acrylic_bottom_v20 (Autodesk Fusion 360 design; units mm, degrees)
Autodesk Fusion 360 part; units mm, degrees
sketch "Sketch1" plane through (0, 0, 0) normal (0, 1, 0) x (1, 0, 0)
  line L0 (193.9, 118.363) -> (193.9, 201.7255) construction
  line L1 (23, 201.7255) -> (23, 118.363) construction
  line L2 (23, 12) -> (193.9, 12) construction
  circle A0 centre (23, 12) radius 1.5
  circle A1 centre (238.9, 12) radius 1.5
  line L3 (193.9, 95.3625) -> (23, 95.3625) construction
  circle A2 centre (238.9, 95.3625) radius 1.5
  circle A3 centre (23, 201.7255) radius 1.5
  line L4 (0, 212.7255) -> (0, 106.363) construction
  circle A4 centre (23, 118.363) radius 1.5
  circle A5 centre (193.9, 201.7255) radius 1.5
  circle A6 centre (23, 95.3625) radius 1.5
  line L5 (0, 106.3625) -> (0, 0) construction
  circle A7 centre (193.9, 95.3625) radius 1.5
  line L6 (23, 118.363) -> (193.9, 118.363) construction
  line L7 (193.9, 12) -> (193.9, 95.3625) construction
  circle A8 centre (193.9, 118.363) radius 1.5
  circle A9 centre (193.9, 12) radius 1.5
  line L8 (215.9, 0) -> (215.9, 106.3625) construction
  circle A10 centre (409.8, 118.363) radius 1.5
  line L9 (238.9, 118.363) -> (409.8, 118.363) construction
  line L10 (23, 95.3625) -> (23, 12) construction
  line L11 (215.9, 0) -> (431.8, 0) construction
  line L12 (431.8, 0) -> (431.8, 106.3625) construction
  line L13 (0, 106.363) -> (215.9, 106.363) construction
  circle A11 centre (409.8, 201.7255) radius 1.5
  line L14 (215.9, 106.3625) -> (0, 106.3625) construction
  line L15 (409.8, 201.7255) -> (238.9, 201.7255) construction
  line L16 (409.8, 12) -> (409.8, 95.3625) construction
  line L17 (215.9, 212.7255) -> (0, 212.7255) construction
  line L18 (0, 0) -> (215.9, 0) construction
  line L19 (215.9, 106.3625) -> (215.9, 0) construction
  circle A12 centre (409.8, 12) radius 1.5
  line L20 (215.9, 106.363) -> (431.8, 106.363) construction
  line L21 (409.8, 118.363) -> (409.8, 201.7255) construction
  line L22 (215.9, 106.363) -> (215.9, 212.7255) construction
  line L23 (238.9, 95.3625) -> (238.9, 12) construction
  circle A13 centre (409.8, 95.3625) radius 1.5
  line L24 (238.9, 12) -> (409.8, 12) construction
  line L25 (431.8, 106.363) -> (431.8, 212.7255) construction
  line L26 (431.8, 212.7255) -> (215.9, 212.7255) construction
  line L27 (409.8, 95.3625) -> (238.9, 95.3625) construction
  line L28 (193.9, 201.7255) -> (23, 201.7255) construction
  line L29 (431.8, 106.3625) -> (215.9, 106.3625) construction
  circle A14 centre (238.9, 118.363) radius 1.5
  circle A15 centre (238.9, 201.7255) radius 1.5
  line L30 (238.9, 201.7255) -> (238.9, 118.363) construction
  line L31 (215.9, 212.7255) -> (215.9, 106.363) construction
  line L32 (432.8, 122.8753) -> (432.8, 213.7255)
  line L33 (432.8, 213.7255) -> (215.9, 213.7255)
  line L34 (215.9, 213.7255) -> (-1, 213.7255)
  line L35 (-1, 213.7255) -> (-1, 97.8373)
  line L36 (-1, 97.8373) -> (-1, -1)
  line L37 (-1, -1) -> (215.9, -1)
  line L38 (215.9, -1) -> (432.8, -1)
  line L39 (432.8, -1) -> (432.8, 122.8753)
  point P0 (215.9, 106.363)
  point P1 (0, 106.363)
  point P2 (215.9, 0)
  dimension "d3" = 215.9
  dimension "d4" = 106.363
  dimension "d5" = 106.3625
  dimension "d6" = 215.9
  dimension "d7" = 23
  dimension "d8" = 11
  dimension "d9" = 12
  dimension "d10" = 22
  dimension "d11" = 3
  dimension "d12" = 3
  dimension "d13" = 3
  dimension "d14" = 3
  dimension "d23" = 1
  dimension "d24" = 1
  constraint horizontal L18
  constraint vertical L8
  constraint horizontal L14
  constraint vertical L5
  constraint coincident L5.end L18.start
  constraint horizontal L2
  constraint vertical L7
  constraint horizontal L3
  constraint vertical L10
  constraint coincident L3.end A6.centre
  constraint coincident L2.start A0.centre
  constraint coincident L2.end L7.start
  constraint coincident L3.start A7.centre
  constraint coincident L35.end L36.start
  constraint coincident L32.start L39.end
  measures "d5" distance of L5.start L5.end
  measures "d6" distance of P2 L5.end
  measures "d7" distance of L5 L10
  measures "d8" distance of L3 L14
  measures "d9" distance of L2 L18
  measures "d10" distance of L7 L8
  measures "d11" diameter of A6
  measures "d12" diameter of A0
  measures "d13" diameter of A7
  measures "d14" diameter of A9
extrude "Extrude1" add sketch "Sketch1" along normal blind 5.4
sketch "Sketch2" plane through (0, 5.4, 0) normal (0, 1, 0) x (-1, 0, 0)
  circle A0 centre (-409.8, -12) radius 1.5
  circle A1 centre (-23, -95.3625) radius 1.5
  circle A2 centre (-409.8, -201.7255) radius 1.5
  circle A3 centre (-409.8, -95.3625) radius 1.5
  circle A4 centre (-238.9, -118.363) radius 1.5
  circle A5 centre (-238.9, -201.7255) radius 1.5
  circle A6 centre (-23, -12) radius 1.5
  circle A7 centre (-193.9, -201.7255) radius 1.5
  circle A8 centre (-193.9, -95.3625) radius 1.5
  circle A9 centre (-23, -201.7255) radius 1.5
  circle A10 centre (-23, -118.363) radius 1.5
  circle A11 centre (-238.9, -12) radius 1.5
  circle A12 centre (-238.9, -95.3625) radius 1.5
  circle A13 centre (-193.9, -118.363) radius 1.5
  circle A14 centre (-409.8, -118.363) radius 1.5
  circle A15 centre (-193.9, -12) radius 1.5
  line L0 (-432.8, 1) -> (-432.8, -122.8753)
  line L1 (-432.8, -122.8753) -> (-432.8, -213.7255)
  line L2 (-432.8, -213.7255) -> (1, -213.7255)
  line L3 (1, -213.7255) -> (1, -97.8373)
  line L4 (1, -97.8373) -> (1, 1)
  line L5 (1, 1) -> (-432.8, 1)
  line L6 (-399.8, -24) -> (-432.8, -24)
  line L7 (-432.8, -24) -> (-432.8, -84)
  line L8 (-432.8, -84) -> (-399.8, -84)
  line L9 (-399.8, -84) -> (-399.8, -24)
  dimension "d27" = 60
  constraint horizontal L6
  constraint vertical L7
  constraint horizontal L8
  constraint vertical L9
  constraint coincident L0.start L7
  measures "d27" distance of L6.start L8.end
sketch "Sketch3" plane through (0, 5.4, 0) normal (0, 1, 0) x (-1, 0, 0)
  circle A0 centre (-193.9, -12) radius 1.5
  circle A1 centre (-409.8, -118.363) radius 1.5
  circle A2 centre (-193.9, -118.363) radius 1.5
  circle A3 centre (-238.9, -95.3625) radius 1.5
  circle A4 centre (-238.9, -12) radius 1.5
  circle A5 centre (-23, -118.363) radius 1.5
  circle A6 centre (-23, -201.7255) radius 1.5
  line L0 (-432.8, -122.8753) -> (-432.8, -213.7255)
  line L1 (-432.8, -213.7255) -> (1, -213.7255)
  line L2 (1, -213.7255) -> (1, -97.8373)
  line L3 (1, -97.8373) -> (1, 1)
  line L4 (1, 1) -> (-432.8, 1)
  line L5 (-432.8, 1) -> (-432.8, -122.8753)
  circle A7 centre (-193.9, -95.3625) radius 1.5
  circle A8 centre (-193.9, -201.7255) radius 1.5
  circle A9 centre (-23, -12) radius 1.5
  circle A10 centre (-238.9, -201.7255) radius 1.5
  circle A11 centre (-238.9, -118.363) radius 1.5
  circle A12 centre (-409.8, -95.3625) radius 1.5
  circle A13 centre (-409.8, -201.7255) radius 1.5
  circle A14 centre (-23, -95.3625) radius 1.5
  circle A15 centre (-409.8, -12) radius 1.5
  line L6 (1, -213.7255) -> (6.4, -213.7255)
  line L7 (6.4, -213.7255) -> (6.4, -193.7255)
  line L8 (6.4, -193.7255) -> (1, -193.7255)
  line L9 (1, -193.7255) -> (1, -213.7255)
  line L10 (1, 1) -> (6.4, 1)
  line L11 (6.4, 1) -> (6.4, -19)
  line L12 (6.4, -19) -> (1, -19)
  line L13 (1, -19) -> (1, 1)
  line L14 (1, 1) -> (-19, 1)
  line L15 (-19, 1) -> (-19, 6.4)
  line L16 (-19, 6.4) -> (1, 6.4)
  line L17 (1, 6.4) -> (1, 1)
  line L18 (1, -213.7255) -> (-19, -213.7255)
  line L19 (-19, -213.7255) -> (-19, -219.1255)
  line L20 (-19, -219.1255) -> (1, -219.1255)
  line L21 (1, -219.1255) -> (1, -213.7255)
  line L22 (-432.8, -213.7255) -> (-412.8, -213.7255)
  line L23 (-412.8, -213.7255) -> (-412.8, -219.1255)
  line L24 (-412.8, -219.1255) -> (-432.8, -219.1255)
  line L25 (-432.8, -219.1255) -> (-432.8, -213.7255)
  line L26 (-432.8, -213.7255) -> (-438.2, -213.7255)
  line L27 (-438.2, -213.7255) -> (-438.2, -193.7255)
  line L28 (-438.2, -193.7255) -> (-432.8, -193.7255)
  line L29 (-432.8, -193.7255) -> (-432.8, -213.7255)
  line L30 (-432.8, 1) -> (-438.2, 1)
  line L31 (-438.2, 1) -> (-438.2, -19)
  line L32 (-438.2, -19) -> (-432.8, -19)
  line L33 (-432.8, -19) -> (-432.8, 1)
  line L34 (-432.8, 1) -> (-412.8, 1)
  line L35 (-412.8, 1) -> (-412.8, 6.4)
  line L36 (-412.8, 6.4) -> (-432.8, 6.4)
  line L37 (-432.8, 6.4) -> (-432.8, 1)
  line L38 (-205.9, 1) -> (-225.9, 1)
  line L39 (-225.9, 1) -> (-225.9, 6.4)
  line L40 (-225.9, 6.4) -> (-205.9, 6.4)
  line L41 (-205.9, 6.4) -> (-205.9, 1)
  line L42 (-205.9, -213.7255) -> (-225.9, -213.7255)
  line L43 (-225.9, -213.7255) -> (-225.9, -219.1255)
  line L44 (-225.9, -219.1255) -> (-205.9, -219.1255)
  line L45 (-205.9, -219.1255) -> (-205.9, -213.7255)
  dimension "d30" = 5.4
  dimension "d31" = 20
  dimension "d32" = 5.4
  dimension "d33" = 20
  dimension "d34" = 20
  dimension "d35" = 5.4
  dimension "d36" = 5.4
  dimension "d37" = 20
  dimension "d38" = 20
  dimension "d39" = 5.4
  dimension "d40" = 5.4
  dimension "d41" = 20
  dimension "d42" = 5.4
  dimension "d43" = 20
  dimension "d44" = 20
  dimension "d45" = 5.4
  dimension "d46" = 20
  dimension "d47" = 5.4
  dimension "d48" = 20
  dimension "d49" = 5.4
  dimension "d50" = 206.9
  dimension "d51" = 206.9
  dimension "d65" = 433.8
  constraint horizontal L6
  constraint vertical L7
  constraint horizontal L8
  constraint vertical L9
  constraint coincident L1.end L2.start
  constraint horizontal L10
  constraint vertical L11
  constraint horizontal L12
  constraint vertical L13
  constraint coincident L3.end L4.start
  constraint horizontal L14
  constraint vertical L15
  constraint horizontal L16
  constraint vertical L17
  constraint horizontal L18
  constraint vertical L19
  constraint horizontal L20
  constraint vertical L21
  constraint horizontal L22
  constraint vertical L23
  constraint horizontal L24
  constraint vertical L25
  constraint coincident L0.end L1.start
  constraint horizontal L26
  constraint vertical L27
  constraint horizontal L28
  constraint vertical L29
  constraint horizontal L30
  constraint vertical L31
  constraint horizontal L32
  constraint vertical L33
  constraint coincident L4.end L5.start
  constraint horizontal L34
  constraint vertical L35
  constraint horizontal L36
  constraint vertical L37
  constraint horizontal L38
  constraint vertical L39
  constraint horizontal L40
  constraint vertical L41
  constraint coincident L4 L38.start
  constraint horizontal L42
  constraint vertical L43
  constraint horizontal L44
  constraint vertical L45
  constraint coincident L1 L42.start
  measures "d30" distance of L3.end L10.end
  measures "d31" distance of L10.end L11.end
  measures "d32" distance of L1.end L6.end
  measures "d33" distance of L6.end L7.end
  measures "d34" distance of L3.end L14.end
  measures "d35" distance of L3.end L16.end
  measures "d36" distance of L1.end L20.end
  measures "d37" distance of L19.end L20.end
  measures "d38" distance of L0.end L22.end
  measures "d39" distance of L0.end L24.end
  measures "d40" distance of L0.end L26.end
  measures "d41" distance of L0.end L28.end
  measures "d42" distance of L4.end L30.end
  measures "d43" distance of L4.end L32.end
  measures "d44" distance of L4.end L34.end
  measures "d45" distance of L4.end L36.end
  measures "d46" distance of L38.start L38.end
  measures "d47" distance of L38.start L40.end
  measures "d48" distance of L42.start L42.end
  measures "d49" distance of L42.start L44.end
  measures "d50" distance of L2 L45
  measures "d51" distance of L3 L41
  measures "d65" distance of L0 L2
extrude "Extrude3" add sketch "Sketch3" against normal blind 5.4 contours L0 L26 L27 L28 L29 | L5 L30 L31 L32 L33 | L1 L22 L23 L24 L25 | L4 L34 L35 L36 L37 | L1 L42 L43 L44 L45 | L4 L38 L39 L40 L41 | L1 L18 L19 L20 L21 | L4 L14 L15 L16 L17 | L2 L6 L7 L8 L9 | L3 L10 L11 L12 L13
sketch "Sketch4" plane through (0, 5.4, 0) normal (0, 1, 0) x (-1, 0, 0)
  circle A0 centre (-238.9, -118.363) radius 1.5
  circle A1 centre (-238.9, -95.3625) radius 1.5
  circle A2 centre (-409.8, -95.3625) radius 1.5
  circle A3 centre (-238.9, -201.7255) radius 1.5
  circle A4 centre (-23, -201.7255) radius 1.5
  circle A5 centre (-409.8, -12) radius 1.5
  circle A6 centre (-193.9, -201.7255) radius 1.5
  circle A7 centre (-238.9, -12) radius 1.5
  circle A8 centre (-23, -118.363) radius 1.5
  circle A9 centre (-23, -12) radius 1.5
  circle A10 centre (-193.9, -95.3625) radius 1.5
  circle A11 centre (-23, -95.3625) radius 1.5
  circle A12 centre (-409.8, -118.363) radius 1.5
  circle A13 centre (-193.9, -12) radius 1.5
  circle A14 centre (-409.8, -201.7255) radius 1.5
  circle A15 centre (-193.9, -118.363) radius 1.5
  line L0 (-432.8, -19) -> (-432.8, -122.8753)
  line L1 (-432.8, -122.8753) -> (-432.8, -193.7255)
  line L2 (-432.8, -193.7255) -> (-438.2, -193.7255)
  line L3 (-438.2, -193.7255) -> (-438.2, -213.7255)
  line L4 (-438.2, -213.7255) -> (-432.8, -213.7255)
  line L5 (-432.8, -213.7255) -> (-432.8, -219.1255)
  line L6 (-432.8, -219.1255) -> (-412.8, -219.1255)
  line L7 (-412.8, -219.1255) -> (-412.8, -213.7255)
  line L8 (-412.8, -213.7255) -> (-225.9, -213.7255)
  line L9 (-225.9, -213.7255) -> (-225.9, -219.1255)
  line L10 (-225.9, -219.1255) -> (-205.9, -219.1255)
  line L11 (-205.9, -219.1255) -> (-205.9, -213.7255)
  line L12 (-205.9, -213.7255) -> (-19, -213.7255)
  line L13 (-19, -213.7255) -> (-19, -219.1255)
  line L14 (-19, -219.1255) -> (1, -219.1255)
  line L15 (1, -219.1255) -> (1, -213.7255)
  line L16 (1, -213.7255) -> (6.4, -213.7255)
  line L17 (6.4, -213.7255) -> (6.4, -193.7255)
  line L18 (6.4, -193.7255) -> (1, -193.7255)
  line L19 (1, -193.7255) -> (1, -97.8373)
  line L20 (1, -97.8373) -> (1, -19)
  line L21 (1, -19) -> (6.4, -19)
  line L22 (6.4, -19) -> (6.4, 1)
  line L23 (6.4, 1) -> (1, 1)
  line L24 (1, 1) -> (1, 6.4)
  line L25 (1, 6.4) -> (-19, 6.4)
  line L26 (-19, 6.4) -> (-19, 1)
  line L27 (-19, 1) -> (-205.9, 1)
  line L28 (-205.9, 1) -> (-205.9, 6.4)
  line L29 (-205.9, 6.4) -> (-225.9, 6.4)
  line L30 (-225.9, 6.4) -> (-225.9, 1)
  line L31 (-225.9, 1) -> (-412.8, 1)
  line L32 (-412.8, 1) -> (-412.8, 6.4)
  line L33 (-412.8, 6.4) -> (-432.8, 6.4)
  line L34 (-432.8, 6.4) -> (-432.8, 1)
  line L35 (-432.8, 1) -> (-438.2, 1)
  line L36 (-438.2, 1) -> (-438.2, -19)
  line L37 (-438.2, -19) -> (-432.8, -19)
  line L38 (6.4, -116.3627) -> (1, -116.3627)
  line L39 (1, -116.3627) -> (1, -96.3627)
  line L40 (1, -96.3627) -> (6.4, -96.3627)
  line L41 (6.4, -96.3627) -> (6.4, -116.3627)
  line L42 (-432.8, -116.3627) -> (-438.2, -116.3627)
  line L43 (-438.2, -116.3627) -> (-438.2, -96.3627)
  line L44 (-438.2, -96.3627) -> (-432.8, -96.3627)
  line L45 (-432.8, -96.3627) -> (-432.8, -116.3627)
  dimension "d54" = 5.4
  dimension "d55" = 20
  dimension "d56" = 174.7255
  dimension "d57" = 77.3628
  dimension "d60" = 5.4
  dimension "d61" = 20
  dimension "d62" = 77.3628
  dimension "d125" = 20
  dimension "d126" = 5.4
  constraint horizontal L38
  constraint vertical L39
  constraint horizontal L40
  constraint vertical L41
  constraint coincident L19 L38.end
  constraint horizontal L42
  constraint vertical L43
  constraint horizontal L44
  constraint vertical L45
  constraint coincident L0 L42.start
  measures "d54" distance of L38.start L38.end
  measures "d55" distance of L38.start L40.end
  measures "d56" distance of L18.end L20.end
  measures "d57" distance of L20.end L39.end
  measures "d60" distance of L42.start L42.end
  measures "d61" distance of L42.start L44.end
  measures "d62" distance of L37 L44
  measures "d125" distance of L16.end L17.end
  measures "d126" distance of L15.end L16.end
extrude "Extrude4" add sketch "Sketch4" against normal blind 5.4 contours L0 L42 L43 L44 L45 | L19 L20 L38 L39 L40 L41
sketch "Sketch5" plane through (0, 5.4, 0) normal (0, 1, 0) x (-1, 0, 0)
  circle A0 centre (-409.8, -95.3625) radius 1.5
  circle A1 centre (-238.9, -201.7255) radius 1.5
  circle A2 centre (-23, -201.7255) radius 1.5
  circle A3 centre (-409.8, -12) radius 1.5
  circle A4 centre (-193.9, -201.7255) radius 1.5
  circle A5 centre (-409.8, -118.363) radius 1.5
  circle A6 centre (-409.8, -201.7255) radius 1.5
  line L0 (-432.8, -19) -> (-432.8, -96.3627)
  line L1 (-432.8, -96.3627) -> (-438.2, -96.3627)
  line L2 (-438.2, -96.3627) -> (-438.2, -116.3627)
  line L3 (-438.2, -116.3627) -> (-432.8, -116.3627)
  line L4 (-432.8, -116.3627) -> (-432.8, -122.8753)
  line L5 (-432.8, -122.8753) -> (-432.8, -193.7255)
  line L6 (-432.8, -193.7255) -> (-438.2, -193.7255)
  line L7 (-438.2, -193.7255) -> (-438.2, -213.7255)
  line L8 (-438.2, -213.7255) -> (-432.8, -213.7255)
  line L9 (-432.8, -213.7255) -> (-432.8, -219.1255)
  line L10 (-432.8, -219.1255) -> (-412.8, -219.1255)
  line L11 (-412.8, -219.1255) -> (-412.8, -213.7255)
  line L12 (-412.8, -213.7255) -> (-225.9, -213.7255)
  line L13 (-225.9, -213.7255) -> (-225.9, -219.1255)
  line L14 (-225.9, -219.1255) -> (-205.9, -219.1255)
  line L15 (-205.9, -219.1255) -> (-205.9, -213.7255)
  line L16 (-205.9, -213.7255) -> (-19, -213.7255)
  line L17 (-19, -213.7255) -> (-19, -219.1255)
  line L18 (-19, -219.1255) -> (1, -219.1255)
  line L19 (1, -219.1255) -> (1, -213.7255)
  line L20 (1, -213.7255) -> (6.4, -213.7255)
  line L21 (6.4, -213.7255) -> (6.4, -193.7255)
  line L22 (6.4, -193.7255) -> (1, -193.7255)
  line L23 (1, -193.7255) -> (1, -116.3627)
  line L24 (1, -116.3627) -> (6.4, -116.3627)
  line L25 (6.4, -116.3627) -> (6.4, -96.3627)
  line L26 (6.4, -96.3627) -> (1, -96.3627)
  line L27 (1, -96.3627) -> (1, -19)
  line L28 (1, -19) -> (6.4, -19)
  line L29 (6.4, -19) -> (6.4, 1)
  line L30 (6.4, 1) -> (1, 1)
  line L31 (1, 1) -> (1, 6.4)
  line L32 (1, 6.4) -> (-19, 6.4)
  line L33 (-19, 6.4) -> (-19, 1)
  line L34 (-19, 1) -> (-205.9, 1)
  line L35 (-205.9, 1) -> (-205.9, 6.4)
  line L36 (-205.9, 6.4) -> (-225.9, 6.4)
  line L37 (-225.9, 6.4) -> (-225.9, 1)
  line L38 (-225.9, 1) -> (-412.8, 1)
  line L39 (-412.8, 1) -> (-412.8, 6.4)
  line L40 (-412.8, 6.4) -> (-432.8, 6.4)
  line L41 (-432.8, 6.4) -> (-432.8, 1)
  line L42 (-432.8, 1) -> (-438.2, 1)
  line L43 (-438.2, 1) -> (-438.2, -19)
  line L44 (-438.2, -19) -> (-432.8, -19)
  line L45 (-360.5, -52.6814) -> (-71.3, -52.6814) construction
  line L46 (-71.3, -160.0441) -> (-360.5, -160.0441) construction
  line L47 (-71.3, -52.6814) -> (-71.3, -160.0441) construction
  circle A7 centre (-71.3, -160.0441) radius 4.445
  line L48 (-73.1415, -150.8366) -> (-73.1415, -169.2516)
  arc A8 (-73.1415, -169.2516) -> (-69.4585, -169.2516) centre (-71.3, -169.2516) ccw
  line L49 (-69.4585, -169.2516) -> (-69.4585, -150.8366)
  arc A9 (-69.4585, -150.8366) -> (-73.1415, -150.8366) centre (-71.3, -150.8366) ccw
  line L50 (-71.3, -150.8366) -> (-71.3, -169.2516) construction
  line L51 (-80.5075, -161.8856) -> (-62.0925, -161.8856)
  arc A10 (-62.0925, -161.8856) -> (-62.0925, -158.2026) centre (-62.0925, -160.0441) ccw
  line L52 (-62.0925, -158.2026) -> (-80.5075, -158.2026)
  arc A11 (-80.5075, -158.2026) -> (-80.5075, -161.8856) centre (-80.5075, -160.0441) ccw
  line L53 (-80.5075, -160.0441) -> (-62.0925, -160.0441) construction
  line L54 (-369.7075, -161.8856) -> (-351.2925, -161.8856)
  arc A12 (-362.3415, -169.2516) -> (-358.6585, -169.2516) centre (-360.5, -169.2516) ccw
  arc A13 (-351.2925, -161.8856) -> (-351.2925, -158.2026) centre (-351.2925, -160.0441) ccw
  arc A14 (-369.7075, -158.2026) -> (-369.7075, -161.8856) centre (-369.7075, -160.0441) ccw
  line L55 (-358.6585, -169.2516) -> (-358.6585, -150.8366)
  circle A15 centre (-360.5, -160.0441) radius 4.445
  line L56 (-362.3415, -150.8366) -> (-362.3415, -169.2516)
  arc A16 (-358.6585, -150.8366) -> (-362.3415, -150.8366) centre (-360.5, -150.8366) ccw
  line L57 (-351.2925, -158.2026) -> (-369.7075, -158.2026)
  line L58 (-360.5, -150.8366) -> (-360.5, -169.2516) construction
  line L59 (-369.7075, -160.0441) -> (-351.2925, -160.0441) construction
  line L60 (-360.5, -52.6814) -> (-360.5, -160.0441) construction
  line L61 (-360.5, -43.4739) -> (-360.5, -61.8889) construction
  arc A17 (-362.3415, -61.8889) -> (-358.6585, -61.8889) centre (-360.5, -61.8889) ccw
  line L62 (-351.2925, -50.8399) -> (-369.7075, -50.8399)
  line L63 (-369.7075, -52.6814) -> (-351.2925, -52.6814) construction
  line L64 (-362.3415, -43.4739) -> (-362.3415, -61.8889)
  arc A18 (-358.6585, -43.4739) -> (-362.3415, -43.4739) centre (-360.5, -43.4739) ccw
  line L65 (-369.7075, -54.5229) -> (-351.2925, -54.5229)
  line L66 (-358.6585, -61.8889) -> (-358.6585, -43.4739)
  circle A19 centre (-360.5, -52.6814) radius 4.445
  arc A20 (-369.7075, -50.8399) -> (-369.7075, -54.5229) centre (-369.7075, -52.6814) ccw
  arc A21 (-351.2925, -54.5229) -> (-351.2925, -50.8399) centre (-351.2925, -52.6814) ccw
  line L67 (-71.3, -43.4739) -> (-71.3, -61.8889) construction
  arc A22 (-73.1415, -61.8889) -> (-69.4585, -61.8889) centre (-71.3, -61.8889) ccw
  line L68 (-62.0925, -50.8399) -> (-80.5075, -50.8399)
  line L69 (-80.5075, -52.6814) -> (-62.0925, -52.6814) construction
  line L70 (-73.1415, -43.4739) -> (-73.1415, -61.8889)
  arc A23 (-69.4585, -43.4739) -> (-73.1415, -43.4739) centre (-71.3, -43.4739) ccw
  line L71 (-80.5075, -54.5229) -> (-62.0925, -54.5229)
  line L72 (-69.4585, -61.8889) -> (-69.4585, -43.4739)
  circle A24 centre (-71.3, -52.6814) radius 4.445
  arc A25 (-80.5075, -50.8399) -> (-80.5075, -54.5229) centre (-80.5075, -52.6814) ccw
  arc A26 (-62.0925, -54.5229) -> (-62.0925, -50.8399) centre (-62.0925, -52.6814) ccw
  point P0 (-71.3, -160.0441)
  point P1 (-71.3, -160.0441)
  point P2 (-360.5, -160.0441)
  point P3 (-360.5, -160.0441)
  point P4 (-360.5, -52.6814)
  point P5 (-360.5, -52.6814)
  point P6 (-360.5, -52.6814)
  point P7 (-360.5, -52.6814)
  point P8 (-71.3, -52.6814)
  point P9 (-71.3, -52.6814)
  point P10 (-71.3, -52.6814)
  point P11 (-71.3, -52.6814)
  dimension "d86" = 214.7255
  dimension "d87" = 433.8
  dimension "d88" = 107.3628
  dimension "d89" = 289.2
  dimension "d90" = 72.3
  dimension "d91" = 53.6814
  dimension "d103" = 8.89
  dimension "d104" = 1.8415
  dimension "d105" = 1.8415
  dimension "d106" = 18.415
  dimension "d107" = 18.415
  dimension "d108" = 8.89
  dimension "d109" = 1.8415
  dimension "d110" = 1.8415
  dimension "d111" = 18.415
  dimension "d112" = 18.415
  dimension "d113" = 8.89
  dimension "d114" = 1.8415
  dimension "d115" = 1.8415
  dimension "d116" = 18.415
  dimension "d117" = 18.415
  dimension "d118" = 8.89
  dimension "d119" = 1.8415
  dimension "d120" = 1.8415
  dimension "d121" = 18.415
  dimension "d122" = 18.415
  constraint horizontal L46
  constraint horizontal L45
  constraint vertical L47
  constraint coincident P1 P0
  constraint tangent L48 A8
  constraint tangent A8 L49
  constraint parallel L48 L49
  constraint tangent L49 A9
  constraint tangent L48 A9
  constraint perpendicular L46 L50
  constraint midpoint L50 P1
  constraint tangent L51 A10
  constraint tangent A10 L52
  constraint parallel L51 L52
  constraint tangent L52 A11
  constraint tangent L51 A11
  constraint perpendicular L47 L53
  constraint midpoint L53 P1
  constraint vertical L60
  constraint coincident P3 P2
  constraint tangent A12 L56
  constraint tangent A12 L55
  constraint parallel L55 L56
  constraint tangent L55 A16
  constraint tangent L56 A16
  constraint midpoint P3 L58
  constraint tangent L54 A13
  constraint tangent A13 L57
  constraint parallel L54 L57
  constraint tangent A14 L57
  constraint tangent L54 A14
  constraint perpendicular L59 L60
  constraint midpoint P3 L59
  constraint parallel L58 L60
  constraint coincident P7 P6
  constraint tangent A17 L64
  constraint tangent A17 L66
  constraint parallel L64 L66
  constraint tangent A18 L66
  constraint tangent L64 A18
  constraint midpoint P7 L61
  constraint tangent L65 A21
  constraint tangent L62 A21
  constraint parallel L62 L65
  constraint tangent L62 A20
  constraint tangent L65 A20
  constraint midpoint P7 L63
  constraint coincident P11 P10
  constraint tangent A22 L70
  constraint tangent A22 L72
  constraint parallel L70 L72
  constraint tangent A23 L72
  constraint tangent L70 A23
  constraint midpoint P11 L67
  constraint tangent L71 A26
  constraint tangent L68 A26
  constraint parallel L68 L71
  constraint tangent L68 A25
  constraint tangent L71 A25
  constraint midpoint P11 L69
  constraint collinear L45 L69
  constraint collinear L47 L67
  constraint collinear L60 L61
  constraint collinear L45 L63
  measures "d86" distance of L16 L34
  measures "d87" distance of L5 L23
  measures "d88" distance of L45 L46
  measures "d89" distance of P1 P3
  measures "d90" distance of L23 L47
  measures "d91" distance of L16 L46
  measures "d103" diameter of A7
  measures "d104" radius of A11
  measures "d105" radius of A8
  measures "d106" distance of A11.centre A10.centre
  measures "d107" distance of A9.centre A8.centre
  measures "d108" diameter of A15
  measures "d109" radius of A14
  measures "d110" radius of A12
  measures "d111" distance of A14.centre A13.centre
  measures "d112" distance of A16.centre A12.centre
  measures "d113" diameter of A19
  measures "d114" radius of A20
  measures "d115" radius of A17
  measures "d116" distance of L63.start L63.end
  measures "d117" distance of L61.end L61.start
  measures "d118" diameter of A24
  measures "d119" radius of A25
  measures "d120" radius of A22
  measures "d121" distance of L69.start L69.end
  measures "d122" distance of L67.end L67.start
sketch "Sketch7" plane through (0, 5.4, 0) normal (0, 1, 0) x (-1, 0, 0)
  circle A0 centre (-238.9, -95.3625) radius 1.5
  circle A1 centre (-409.8, -118.363) radius 1.5
  circle A2 centre (-409.8, -201.7255) radius 1.5
  circle A3 centre (-238.9, -12) radius 1.5
  circle A4 centre (-193.9, -12) radius 1.5
  circle A5 centre (-238.9, -201.7255) radius 1.5
  circle A6 centre (-193.9, -118.363) radius 1.5
  circle A7 centre (-409.8, -12) radius 1.5
  circle A8 centre (-409.8, -95.3625) radius 1.5
  circle A9 centre (-238.9, -118.363) radius 1.5
  circle A10 centre (-23, -118.363) radius 1.5
  circle A11 centre (-23, -201.7255) radius 1.5
  circle A12 centre (-23, -95.3625) radius 1.5
  circle A13 centre (-193.9, -201.7255) radius 1.5
  circle A14 centre (-193.9, -95.3625) radius 1.5
  circle A15 centre (-23, -12) radius 1.5
  line L0 (-432.8, -19) -> (-432.8, -96.3627)
  line L1 (-432.8, -96.3627) -> (-438.2, -96.3627)
  line L2 (-438.2, -96.3627) -> (-438.2, -116.3627)
  line L3 (-438.2, -116.3627) -> (-432.8, -116.3627)
  line L4 (-432.8, -116.3627) -> (-432.8, -122.8753)
  line L5 (-432.8, -122.8753) -> (-432.8, -193.7255)
  line L6 (-432.8, -193.7255) -> (-438.2, -193.7255)
  line L7 (-438.2, -193.7255) -> (-438.2, -213.7255)
  line L8 (-438.2, -213.7255) -> (-432.8, -213.7255)
  line L9 (-432.8, -213.7255) -> (-432.8, -219.1255)
  line L10 (-432.8, -219.1255) -> (-412.8, -219.1255)
  line L11 (-412.8, -219.1255) -> (-412.8, -213.7255)
  line L12 (-412.8, -213.7255) -> (-225.9, -213.7255)
  line L13 (-225.9, -213.7255) -> (-225.9, -219.1255)
  line L14 (-225.9, -219.1255) -> (-205.9, -219.1255)
  line L15 (-205.9, -219.1255) -> (-205.9, -213.7255)
  line L16 (-205.9, -213.7255) -> (-19, -213.7255)
  line L17 (-19, -213.7255) -> (-19, -219.1255)
  line L18 (-19, -219.1255) -> (1, -219.1255)
  line L19 (1, -219.1255) -> (1, -213.7255)
  line L20 (1, -213.7255) -> (6.4, -213.7255)
  line L21 (6.4, -213.7255) -> (6.4, -193.7255)
  line L22 (6.4, -193.7255) -> (1, -193.7255)
  line L23 (1, -193.7255) -> (1, -116.3627)
  line L24 (1, -116.3627) -> (6.4, -116.3627)
  line L25 (6.4, -116.3627) -> (6.4, -96.3627)
  line L26 (6.4, -96.3627) -> (1, -96.3627)
  line L27 (1, -96.3627) -> (1, -19)
  line L28 (1, -19) -> (6.4, -19)
  line L29 (6.4, -19) -> (6.4, 1)
  line L30 (6.4, 1) -> (1, 1)
  line L31 (1, 1) -> (1, 6.4)
  line L32 (1, 6.4) -> (-19, 6.4)
  line L33 (-19, 6.4) -> (-19, 1)
  line L34 (-19, 1) -> (-205.9, 1)
  line L35 (-205.9, 1) -> (-205.9, 6.4)
  line L36 (-205.9, 6.4) -> (-225.9, 6.4)
  line L37 (-225.9, 6.4) -> (-225.9, 1)
  line L38 (-225.9, 1) -> (-412.8, 1)
  line L39 (-412.8, 1) -> (-412.8, 6.4)
  line L40 (-412.8, 6.4) -> (-432.8, 6.4)
  line L41 (-432.8, 6.4) -> (-432.8, 1)
  line L42 (-432.8, 1) -> (-438.2, 1)
  line L43 (-438.2, 1) -> (-438.2, -19)
  line L44 (-438.2, -19) -> (-432.8, -19)
  line L45 (-84, -190.7255) -> (-120, -190.7255)
  line L46 (-120, -190.7255) -> (-120, -175.7255)
  line L47 (-120, -175.7255) -> (-84, -175.7255)
  line L48 (-84, -175.7255) -> (-84, -190.7255)
  line L49 (-84, -85.5455) -> (-120, -85.5455)
  line L50 (-120, -85.5455) -> (-120, -70.5455)
  line L51 (-120, -70.5455) -> (-84, -70.5455)
  line L52 (-84, -70.5455) -> (-84, -85.5455)
  dimension "d95" = 23
  dimension "d96" = 38
  dimension "d97" = 85
  dimension "d99" = 128.18
  dimension "d100" = 15
  dimension "d127" = 36
  constraint horizontal L45
  constraint vertical L46
  constraint horizontal L47
  constraint vertical L48
  constraint horizontal L49
  constraint vertical L50
  constraint horizontal L51
  constraint vertical L52
  constraint collinear L48 L52
  constraint collinear L46 L50
  measures "d95" distance of L16 L45
  measures "d96" distance of L16 L47
  measures "d97" distance of L23 L48
  measures "d99" distance of L16 L49
  measures "d100" distance of L49 L51
  measures "d127" distance of L45.start L45.end
extrude "Extrude6" cut sketch "Sketch7" against normal blind 20 contours L45 L46 L47 L48 | L49 L50 L51 L52
extrude "Extrude7" cut sketch "Sketch5" against normal blind 9 contours A7 L49 L51 L52 | A7 L51 A10 L52 | A7 L49 L52 | A7 L49 L51 | A7 L48 L49 L52 | A7 L48 L49 A9 | L48 L49 L51 L52 | A7 L48 A8 L49 | A7 L48 L49 L51 | A7 L48 L52 | A7 L48 L51 L52 | A7 L48 L51 | A7 L51 L52 A11 | L54 A14 A15 L57 | L54 A15 L56 L57 | L54 A15 L56 | L54 L55 L56 L57 | L54 L55 A15 L56 | A15 L56 L57 | A12 L55 A15 L56 | L54 L55 A15 L57 | L54 L55 A15 | L55 A15 L56 L57 | L55 A15 L56 A16 | L54 A13 A15 L57 | L55 A15 L57 | A17 L64 L66 A19 | L64 L65 A19 | L64 L65 L66 A19 | L65 L66 A19 | L62 L64 L65 A19 | L62 L64 L65 L66 | L62 L65 A19 A20 | L62 L65 L66 A19 | L62 L65 A19 A21 | L62 L64 L66 A19 | L62 L64 A19 | L62 L66 A19 | L64 A18 L66 A19 | A22 L70 L72 A24 | L70 L71 A24 | L70 L71 L72 A24 | L71 L72 A24 | L68 L70 L71 A24 | L68 L70 L71 L72 | L68 L71 A24 A25 | L68 L71 L72 A24 | L68 L71 A24 A26 | L68 L70 L72 A24 | L68 L70 A24 | L68 L72 A24 | L70 A23 L72 A24
sketch "export" plane through (0, 5.4, 0) normal (0, 1, 0) x (-1, 0, 0)
  line L0 (-67.2544, -50.8399) -> (-62.0925, -50.8399)
  arc A0 (-62.0925, -54.5229) -> (-62.0925, -50.8399) centre (-62.0925, -52.6814) ccw
  line L1 (-62.0925, -54.5229) -> (-67.2544, -54.5229)
  arc A1 (-69.4585, -56.727) -> (-67.2544, -54.5229) centre (-71.3, -52.6814) ccw
  line L2 (-69.4585, -56.727) -> (-69.4585, -61.8889)
  arc A2 (-73.1415, -61.8889) -> (-69.4585, -61.8889) centre (-71.3, -61.8889) ccw
  line L3 (-73.1415, -61.8889) -> (-73.1415, -56.727)
  arc A3 (-75.3456, -54.5229) -> (-73.1415, -56.727) centre (-71.3, -52.6814) ccw
  line L4 (-75.3456, -54.5229) -> (-80.5075, -54.5229)
  arc A4 (-80.5075, -50.8399) -> (-80.5075, -54.5229) centre (-80.5075, -52.6814) ccw
  line L5 (-80.5075, -50.8399) -> (-75.3456, -50.8399)
  arc A5 (-73.1415, -48.6358) -> (-75.3456, -50.8399) centre (-71.3, -52.6814) ccw
  line L6 (-73.1415, -48.6358) -> (-73.1415, -43.4739)
  arc A6 (-69.4585, -43.4739) -> (-73.1415, -43.4739) centre (-71.3, -43.4739) ccw
  line L7 (-69.4585, -43.4739) -> (-69.4585, -48.6358)
  arc A7 (-67.2544, -50.8399) -> (-69.4585, -48.6358) centre (-71.3, -52.6814) ccw
  line L8 (-356.4544, -50.8399) -> (-351.2925, -50.8399)
  arc A8 (-351.2925, -54.5229) -> (-351.2925, -50.8399) centre (-351.2925, -52.6814) ccw
  line L9 (-351.2925, -54.5229) -> (-356.4544, -54.5229)
  arc A9 (-358.6585, -56.727) -> (-356.4544, -54.5229) centre (-360.5, -52.6814) ccw
  line L10 (-358.6585, -56.727) -> (-358.6585, -61.8889)
  arc A10 (-362.3415, -61.8889) -> (-358.6585, -61.8889) centre (-360.5, -61.8889) ccw
  line L11 (-362.3415, -61.8889) -> (-362.3415, -56.727)
  arc A11 (-364.5456, -54.5229) -> (-362.3415, -56.727) centre (-360.5, -52.6814) ccw
  line L12 (-364.5456, -54.5229) -> (-369.7075, -54.5229)
  arc A12 (-369.7075, -50.8399) -> (-369.7075, -54.5229) centre (-369.7075, -52.6814) ccw
  line L13 (-369.7075, -50.8399) -> (-364.5456, -50.8399)
  arc A13 (-362.3415, -48.6358) -> (-364.5456, -50.8399) centre (-360.5, -52.6814) ccw
  line L14 (-362.3415, -48.6358) -> (-362.3415, -43.4739)
  arc A14 (-358.6585, -43.4739) -> (-362.3415, -43.4739) centre (-360.5, -43.4739) ccw
  line L15 (-358.6585, -43.4739) -> (-358.6585, -48.6358)
  arc A15 (-356.4544, -50.8399) -> (-358.6585, -48.6358) centre (-360.5, -52.6814) ccw
  line L16 (-75.3456, -161.8856) -> (-80.5075, -161.8856)
  arc A16 (-80.5075, -158.2026) -> (-80.5075, -161.8856) centre (-80.5075, -160.0441) ccw
  line L17 (-80.5075, -158.2026) -> (-75.3456, -158.2026)
  arc A17 (-73.1415, -155.9985) -> (-75.3456, -158.2026) centre (-71.3, -160.0441) ccw
  line L18 (-73.1415, -155.9985) -> (-73.1415, -150.8366)
  arc A18 (-69.4585, -150.8366) -> (-73.1415, -150.8366) centre (-71.3, -150.8366) ccw
  line L19 (-69.4585, -150.8366) -> (-69.4585, -155.9985)
  arc A19 (-67.2544, -158.2026) -> (-69.4585, -155.9985) centre (-71.3, -160.0441) ccw
  line L20 (-67.2544, -158.2026) -> (-62.0925, -158.2026)
  arc A20 (-62.0925, -161.8856) -> (-62.0925, -158.2026) centre (-62.0925, -160.0441) ccw
  line L21 (-62.0925, -161.8856) -> (-67.2544, -161.8856)
  arc A21 (-69.4585, -164.0897) -> (-67.2544, -161.8856) centre (-71.3, -160.0441) ccw
  line L22 (-69.4585, -164.0897) -> (-69.4585, -169.2516)
  arc A22 (-73.1415, -169.2516) -> (-69.4585, -169.2516) centre (-71.3, -169.2516) ccw
  line L23 (-73.1415, -169.2516) -> (-73.1415, -164.0897)
  arc A23 (-75.3456, -161.8856) -> (-73.1415, -164.0897) centre (-71.3, -160.0441) ccw
  arc A24 (-356.4544, -158.2026) -> (-358.6585, -155.9985) centre (-360.5, -160.0441) ccw
  line L24 (-356.4544, -158.2026) -> (-351.2925, -158.2026)
  arc A25 (-351.2925, -161.8856) -> (-351.2925, -158.2026) centre (-351.2925, -160.0441) ccw
  line L25 (-351.2925, -161.8856) -> (-356.4544, -161.8856)
  arc A26 (-358.6585, -164.0897) -> (-356.4544, -161.8856) centre (-360.5, -160.0441) ccw
  line L26 (-358.6585, -164.0897) -> (-358.6585, -169.2516)
  arc A27 (-362.3415, -169.2516) -> (-358.6585, -169.2516) centre (-360.5, -169.2516) ccw
  line L27 (-362.3415, -169.2516) -> (-362.3415, -164.0897)
  arc A28 (-364.5456, -161.8856) -> (-362.3415, -164.0897) centre (-360.5, -160.0441) ccw
  line L28 (-364.5456, -161.8856) -> (-369.7075, -161.8856)
  arc A29 (-369.7075, -158.2026) -> (-369.7075, -161.8856) centre (-369.7075, -160.0441) ccw
  line L29 (-369.7075, -158.2026) -> (-364.5456, -158.2026)
  arc A30 (-362.3415, -155.9985) -> (-364.5456, -158.2026) centre (-360.5, -160.0441) ccw
  line L30 (-362.3415, -155.9985) -> (-362.3415, -150.8366)
  arc A31 (-358.6585, -150.8366) -> (-362.3415, -150.8366) centre (-360.5, -150.8366) ccw
  line L31 (-358.6585, -150.8366) -> (-358.6585, -155.9985)
  line L32 (-120, -190.7255) -> (-120, -175.7255)
  line L33 (-120, -175.7255) -> (-84, -175.7255)
  line L34 (-84, -175.7255) -> (-84, -190.7255)
  line L35 (-84, -190.7255) -> (-120, -190.7255)
  line L36 (-120, -85.5455) -> (-120, -70.5455)
  line L37 (-120, -70.5455) -> (-84, -70.5455)
  line L38 (-84, -70.5455) -> (-84, -85.5455)
  line L39 (-84, -85.5455) -> (-120, -85.5455)
  circle A32 centre (-238.9, -95.3625) radius 1.5
  circle A33 centre (-409.8, -118.363) radius 1.5
  circle A34 centre (-409.8, -201.7255) radius 1.5
  circle A35 centre (-238.9, -12) radius 1.5
  circle A36 centre (-193.9, -12) radius 1.5
  circle A37 centre (-238.9, -201.7255) radius 1.5
  circle A38 centre (-193.9, -118.363) radius 1.5
  circle A39 centre (-409.8, -12) radius 1.5
  circle A40 centre (-409.8, -95.3625) radius 1.5
  circle A41 centre (-238.9, -118.363) radius 1.5
  circle A42 centre (-23, -118.363) radius 1.5
  circle A43 centre (-23, -201.7255) radius 1.5
  circle A44 centre (-23, -95.3625) radius 1.5
  circle A45 centre (-193.9, -201.7255) radius 1.5
  circle A46 centre (-193.9, -95.3625) radius 1.5
  circle A47 centre (-23, -12) radius 1.5
  line L40 (-432.8, -19) -> (-432.8, -96.3627)
  line L41 (-432.8, -96.3627) -> (-438.2, -96.3627)
  line L42 (-438.2, -96.3627) -> (-438.2, -116.3627)
  line L43 (-438.2, -116.3627) -> (-432.8, -116.3627)
  line L44 (-432.8, -116.3627) -> (-432.8, -122.8753)
  line L45 (-432.8, -122.8753) -> (-432.8, -193.7255)
  line L46 (-432.8, -193.7255) -> (-438.2, -193.7255)
  line L47 (-438.2, -193.7255) -> (-438.2, -213.7255)
  line L48 (-438.2, -213.7255) -> (-432.8, -213.7255)
  line L49 (-432.8, -213.7255) -> (-432.8, -219.1255)
  line L50 (-432.8, -219.1255) -> (-412.8, -219.1255)
  line L51 (-412.8, -219.1255) -> (-412.8, -213.7255)
  line L52 (-412.8, -213.7255) -> (-225.9, -213.7255)
  line L53 (-225.9, -213.7255) -> (-225.9, -219.1255)
  line L54 (-225.9, -219.1255) -> (-205.9, -219.1255)
  line L55 (-205.9, -219.1255) -> (-205.9, -213.7255)
  line L56 (-205.9, -213.7255) -> (-19, -213.7255)
  line L57 (-19, -213.7255) -> (-19, -219.1255)
  line L58 (-19, -219.1255) -> (1, -219.1255)
  line L59 (1, -219.1255) -> (1, -213.7255)
  line L60 (1, -213.7255) -> (6.4, -213.7255)
  line L61 (6.4, -213.7255) -> (6.4, -193.7255)
  line L62 (6.4, -193.7255) -> (1, -193.7255)
  line L63 (1, -193.7255) -> (1, -116.3627)
  line L64 (1, -116.3627) -> (6.4, -116.3627)
  line L65 (6.4, -116.3627) -> (6.4, -96.3627)
  line L66 (6.4, -96.3627) -> (1, -96.3627)
  line L67 (1, -96.3627) -> (1, -19)
  line L68 (1, -19) -> (6.4, -19)
  line L69 (6.4, -19) -> (6.4, 1)
  line L70 (6.4, 1) -> (1, 1)
  line L71 (1, 1) -> (1, 6.4)
  line L72 (1, 6.4) -> (-19, 6.4)
  line L73 (-19, 6.4) -> (-19, 1)
  line L74 (-19, 1) -> (-205.9, 1)
  line L75 (-205.9, 1) -> (-205.9, 6.4)
  line L76 (-205.9, 6.4) -> (-225.9, 6.4)
  line L77 (-225.9, 6.4) -> (-225.9, 1)
  line L78 (-225.9, 1) -> (-412.8, 1)
  line L79 (-412.8, 1) -> (-412.8, 6.4)
  line L80 (-412.8, 6.4) -> (-432.8, 6.4)
  line L81 (-432.8, 6.4) -> (-432.8, 1)
  line L82 (-432.8, 1) -> (-438.2, 1)
  line L83 (-438.2, 1) -> (-438.2, -19)
  line L84 (-438.2, -19) -> (-432.8, -19)
equation "d11 = d12"
equation "d13 = d11"
equation "d14 = d11"
equation "d30 = d36"
equation "d31 = d33"
equation "d32 = d36"
equation "d34 = d33"
equation "d35 = d36"
equation "d37 = d33"
equation "d38 = d33"
equation "d39 = d36"
equation "d40 = d36"
equation "d41 = d33"
equation "d42 = d36"
equation "d43 = d33"
equation "d44 = d33"
equation "d45 = d36"
equation "d46 = d33"
equation "d47 = d36"
equation "d48 = d33"
equation "d49 = d36"
equation "d50 = ( d65 - d48 ) / 2"
equation "d51 = d50"
equation "d54 = d126"
equation "d55 = d125"
equation "d57 = ( d56 - d55 ) / 2"
equation "d60 = d54"
equation "d61 = d55"
equation "d62 = d57"
equation "d88 = 0.5 * d86"
equation "d89 = 2 * d87 / 3"
equation "d90 = ( d87 - d89 ) / 2"
equation "d91 = ( d86 - d88 ) / 2"
equation "d100 = d96 - d95"
equation "d104 = 0.145 in / 2"
equation "d105 = d104"
equation "d106 = d105 * 10"
equation "d107 = d106"
equation "d109 = 0.145 in / 2"
equation "d110 = d104"
equation "d111 = d105 * 10"
equation "d112 = d106"
equation "d114 = 0.145 in / 2"
equation "d115 = d104"
equation "d116 = d105 * 10"
equation "d117 = d106"
equation "d119 = 0.145 in / 2"
equation "d120 = d104"
equation "d121 = d105 * 10"
equation "d122 = d106"
